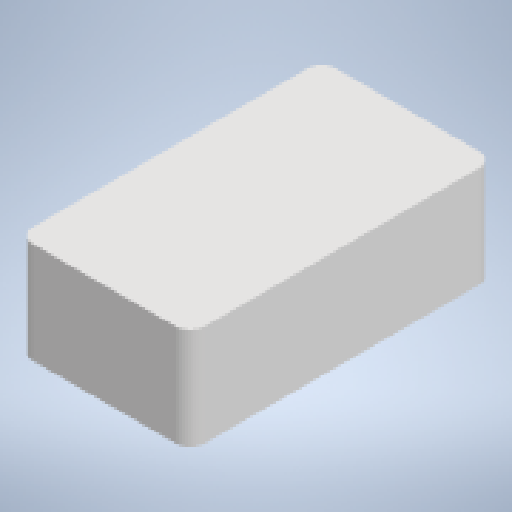
# Autodesk Inventor part: РедукторСмещенный
Saved by Autodesk Inventor 2025.1 (Build 291241000, 241)
## iProperties
Created: 2025-04-12
Part Number: РедукторСмещенный
Material: Типовые
Document SubType Name: Modeling
Designer: tishk
Density: 1 g/cm^3
Appearance: По умолчанию
Author: tishk
Autodesk Inventor part; units mm, degrees
ref_plane "YZ Plane" through (0, 0, 0) normal (1, 0, 0) x (0, 1, 0)
ref_plane "XZ Plane" through (0, 0, 0) normal (0, 1, 0) x (-1, 0, 0)
ref_plane "XY Plane" through (0, 0, 0) normal (0, 0, 1) x (1, 0, 0)
sketch "Эскиз1" plane through (0, 0, 0) normal (0, 1, 0) x (-1, 0, 0)
  line L0 (0, 0) -> (-85, 0)
  line L1 (-85, 0) -> (-85, 150)
  line L2 (-85, 150) -> (0, 150)
  line L3 (0, 150) -> (0, 0)
  dimension "d0" = 85
  dimension "d1" = 150
  constraints: 8 end point, 2 parallel, 1 horizontal, 1 perpendicular
  measures "d0" distance of L1.end L2.end
  measures "d1" distance of L0.end L1.end
extrude "Выдавливание1" add sketch "Эскиз1" along normal blind 50
sketch "Эскиз2" plane through (0, 50, 0) normal (0, 1, 0) x (1, 0, 0)
  line L0 (0, 0) -> (0, -150) projected
  line L1 (0, 0) -> (42.5, 0)
  line L2 (85, 0) -> (0, 0) projected
  line L3 (42.5, 0) -> (42.5, -35)
  dimension "d5" = 42.5
  dimension "d6" = 35
  constraints: 4 end point, 1 midpoint, 1 perpendicular
  measures "d5" distance of L0.start L1.end
  measures "d6" distance of L1.end L3.end
hole "Отверстие1" at (42.5, 50, 35) direction (0, -1, 0) diameter 8 end through all
sketch "Эскиз3" plane through (0, 50, 0) normal (0, 1, 0) x (1, 0, 0)
  line L0 (0, 0) -> (0, -150) projected
  line L1 (0, 0) -> (0, -120)
  line L2 (0, -120) -> (42.5, -120)
  circle A0 centre (42.5, -120) radius 5
  dimension "d14" = 120
  dimension "d15" = 42.5
  dimension "d16" = 10
  constraints: 4 end point, 1 centre point, 1 coincident, 1 perpendicular, 1 point on line
  measures "d14" distance of L0.start L1.end
  measures "d15" distance of L1.end L2.end
  measures "d16" diameter of A0
extrude "Выдавливание2" add sketch "Эскиз3" along normal blind 23.6
fillet "Сопряжение2" radius 7.5 4 edges at (0, 25, 0) (85, 25, 0) (85, 25, 150) (0, 25, 150)
sketch "Эскиз4" plane through (42.5, 73.6, 120) normal (0, 1, 0) x (1, 0, 0)
  circle A0 centre (0, 0) radius 6.154
  point P0 (-42.5, 120)
  dimension "d20" = 12.308
  constraints: 1 centre point
  measures "d20" diameter of A0
extrude "Выдавливание3" add sketch "Эскиз4" along normal blind 46.4
